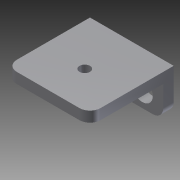
# Autodesk Inventor part: Shooter Curve Support
Saved by Autodesk Inventor 2012 (Build 160160000, 160)
## iProperties
Created: 2013-01-17
Part Number: Shooter Curve Support
Material: Default
Document SubType Name: Modeling
Designer: William
Density: 1 g/cm^3
Mass: 2.56282 g
Surface Area: 21.3848 cm^2
Volume: 2.56282 cm^3
Author: William
Autodesk Inventor part; units mm, degrees
ref_plane "YZ Plane" through (0, 0, 0) normal (1, 0, 0) x (0, 1, 0)
ref_plane "XZ Plane" through (0, 0, 0) normal (0, 1, 0) x (-1, 0, 0)
ref_plane "XY Plane" through (0, 0, 0) normal (0, 0, 1) x (1, 0, 0)
sketch "Sketch1" plane through (0, 0, 0) normal (0, 0, 1) x (1, 0, 0)
  line L0 (-5.1724, -7.3755) -> (20.2276, -7.3755)
  line L1 (20.2276, -7.3755) -> (20.2276, 5.3245)
  line L2 (20.2276, 5.3245) -> (-5.1724, 5.3245)
  line L3 (-5.1724, 5.3245) -> (-5.1724, -7.3755)
  circle A0 centre (1.1776, -2.613) radius 3.175
  circle A1 centre (13.8776, -2.613) radius 3.175
  point P0 (0, 0)
  dimension "d0" = 25.4
  dimension "d1" = 12.7
  dimension "d2" = 6.35
  dimension "d3" = 6.35
  dimension "d5" = 6.35
  dimension "d6" = 6.35
  dimension "d13" = 4.7625
  dimension "d14" = 4.7625
  constraints: 8 end point, 2 centre point, 2 parallel, 1 horizontal, 1 perpendicular
  measures "d0" distance of L2.end L1.end
  measures "d1" distance of L1.end L0.end
  measures "d2" diameter of A0
  measures "d3" diameter of A1
  measures "d5" distance from line of L3 A0.centre
  measures "d6" distance from line of L1 A1.centre
  measures "d13" distance from line of L0 A0.centre
  measures "d14" distance from line of L0 A1.centre
extrude "Extrusion1" add sketch "Sketch1" along normal blind 3.175
sketch "Sketch2" plane through (0, 0, 3.175) normal (0, 0, 1) x (1, 0, 0)
  line L0 (20.2276, 5.3245) -> (20.2276, -7.3755) projected
  line L1 (-5.1724, 5.3245) -> (20.2276, 5.3245) projected
  line L2 (-5.1724, 5.3245) -> (20.2276, 5.3245)
  line L3 (20.2276, 5.3245) -> (20.2276, 2.1495)
  line L4 (20.2276, 2.1495) -> (-5.1724, 2.1495)
  line L5 (-5.1724, 2.1495) -> (-5.1724, 5.3245)
  point P0 (0, 0)
  dimension "d10" = 3.175
  constraints: 8 end point, 2 parallel, 1 horizontal, 1 perpendicular, 1 point on line
  measures "d10" distance of L2.end L3.end
extrude "Extrusion2" add sketch "Sketch2" along normal blind 22.225
sketch "Sketch3" plane through (-5.1724, 2.1495, 3.175) normal (0, -1, 0) x (1, 0, 0)
  circle A0 centre (12.7, 11.1125) radius 1.5875
  point P0 (5.1724, -3.175)
  dimension "d15" = 3.175
  constraints: 1 centre point
  measures "d15" diameter of A0
extrude "Extrusion3" cut sketch "Sketch3" against normal blind 22.225
fillet "Fillet1" radius 3.175 4 edges at (20.2276, 3.737, 25.4) (-5.1724, 3.737, 25.4) (20.2276, -7.3755, 1.5875) (-5.1724, -7.3755, 1.5875)
equation "\"d3\" = d2"
equation "\"d14\" = d13"
body "Solid1"
